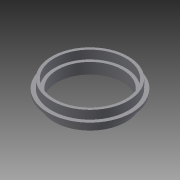
# Autodesk Inventor part: Eyepiece tube filter holder
Saved by Autodesk Inventor 2013 (Build 170138000, 138)
## iProperties
Created: 2013-12-05
Part Number: Eyepiece tube filter holder
Material: Generic
Document SubType Name: Modeling
Designer: kthorn
Density: 1 g/cm^3
Author: kthorn
Autodesk Inventor part; units mm, degrees
ref_plane "YZ Plane" through (0, 0, 0) normal (1, 0, 0) x (0, 1, 0)
ref_plane "XZ Plane" through (0, 0, 0) normal (0, 1, 0) x (-1, 0, 0)
ref_plane "XY Plane" through (0, 0, 0) normal (0, 0, 1) x (1, 0, 0)
sketch "Sketch1" plane through (0, 0, 0) normal (0, 0, 1) x (1, 0, 0)
  circle A0 centre (-3.3222, -5.7216) radius 11.7
  circle A1 centre (-3.3222, -5.7216) radius 12.7
  point P0 (0, 0)
  dimension "d3" = 1
  dimension "d4" = 25.4
  constraints: 2 centre point, 1 coincident
  measures "d3" radial gap between concentric circles of A1 A0
  measures "d4" diameter of A1
extrude "Extrusion1" add sketch "Sketch1" against normal blind 3
sketch "Sketch3" plane through (-3.3222, -5.7216, 0) normal (0, 0, 1) x (1, 0, 0)
  circle A0 centre (0, 0) radius 11.7 projected
  circle A1 centre (0, 0) radius 12.7 projected
  circle A2 centre (0, 0) radius 11.5
  circle A3 centre (0, 0) radius 14.9
  point P0 (3.3222, 5.7216)
  dimension "d12" = 23
  dimension "d14" = 29.8
  constraints: 2 centre point, 2 coincident
  measures "d12" diameter of A2
  measures "d14" diameter of A3
extrude "Extrusion3" add sketch "Sketch3" along normal blind 1 contours A0 | A1 | A3
sketch "Sketch4" plane through (-3.3222, -5.7216, 1) normal (0, 0, 1) x (1, 0, 0)
  circle A0 centre (0, 0) radius 14.9 projected
  circle A1 centre (0, 0) radius 12.6
  circle A2 centre (0, 0) radius 13.6
  point P0 (3.3222, 5.7216)
  dimension "d17" = 1
  dimension "d19" = 25.2
  constraints: 2 centre point, 2 coincident
  measures "d17" radial gap between concentric circles of A2 A1
  measures "d19" diameter of A1
extrude "Extrusion4" add sketch "Sketch4" along normal blind 3 contours A2
body "Solid1"
